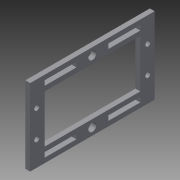
# Autodesk Inventor part: Motor_Mount_Side
Saved by Autodesk Inventor 2014 SP1 (Build 180222100, 222)
## iProperties
Created: 2014-03-20
Part Number: Motor_Mount_Side
Material: Generic
Document SubType Name: Modeling
Designer: ehagerup
Density: 1 g/cm^3
Appearance: Default
Author: ehagerup
Autodesk Inventor part; units mm, degrees
ref_plane "YZ Plane" through (0, 0, 0) normal (1, 0, 0) x (0, 1, 0)
ref_plane "XZ Plane" through (0, 0, 0) normal (0, 1, 0) x (-1, 0, 0)
ref_plane "XY Plane" through (0, 0, 0) normal (0, 0, 1) x (1, 0, 0)
sketch "Sketch1" plane through (0, 0, 0) normal (1, 0, 0) x (0, 1, 0)
  line L0 (0, 0) -> (60, 0)
  line L1 (60, 0) -> (60, 30)
  line L2 (60, 30) -> (0, 30)
  line L3 (0, 30) -> (0, 0)
  line L4 (-9, -9) -> (69, -9)
  line L5 (69, -9) -> (69, 39)
  line L6 (69, 39) -> (-9, 39)
  line L7 (-9, 39) -> (-9, -9)
  circle A0 centre (64.8, 23.5) radius 1.6
  circle A1 centre (64.8, 6.5) radius 1.6
  circle A2 centre (-4.8, 23.5) radius 1.6
  circle A3 centre (-4.8, 6.5) radius 1.6
  line L8 (0, 33) -> (20, 33)
  line L9 (20, 33) -> (20, 36)
  line L10 (20, 36) -> (0, 36)
  line L11 (0, 36) -> (0, 33)
  line L12 (60, 33) -> (40, 33)
  line L13 (40, 33) -> (40, 36)
  line L14 (40, 36) -> (60, 36)
  line L15 (60, 36) -> (60, 33)
  circle A4 centre (30, 34.5) radius 2.5
  circle A5 centre (30, -4.5) radius 2.5
  line L16 (0, -3) -> (20, -3)
  line L17 (20, -3) -> (20, -6)
  line L18 (20, -6) -> (0, -6)
  line L19 (0, -6) -> (0, -3)
  line L20 (60, -3) -> (40, -3)
  line L21 (40, -3) -> (40, -6)
  line L22 (40, -6) -> (60, -6)
  line L23 (60, -6) -> (60, -3)
  dimension "d0" = 60
  dimension "d1" = 30
  dimension "d2" = 4.8
  dimension "d3" = 4.8
  dimension "d4" = 4.8
  dimension "d5" = 4.8
  dimension "d6" = 3.2
  dimension "d7" = 3.2
  dimension "d8" = 3.2
  dimension "d9" = 3.2
  dimension "d10" = 6.5
  dimension "d11" = 6.5
  dimension "d12" = 6.5
  dimension "d13" = 6.5
  dimension "d14" = 9
  dimension "d15" = 9
  dimension "d16" = 9
  dimension "d17" = 9
  dimension "d18" = 20
  dimension "d19" = 9
  dimension "d20" = 3
  dimension "d21" = 3
  dimension "d22" = 9
  dimension "d23" = 3
  dimension "d24" = 3
  dimension "d25" = 20
  dimension "d26" = 5
  dimension "d27" = 10
  dimension "d28" = 4.5
  dimension "d29" = 4.5
  dimension "d30" = 5
  dimension "d31" = 3
  dimension "d32" = 3
  dimension "d33" = 20
  dimension "d34" = 9
  dimension "d35" = 10
  dimension "d36" = 10
  dimension "d37" = 20
  dimension "d38" = 3
  dimension "d39" = 3
  constraints: 48 end point, 12 parallel, 6 centre point, 6 horizontal, 6 perpendicular
  measures "d0" distance of L1.end L2.end
  measures "d1" distance of L0.end L1.end
  measures "d2" distance from line of A1.centre L1
  measures "d3" distance from line of A0.centre L1
  measures "d4" distance from line of L3 A2.centre
  measures "d5" distance from line of L3 A3.centre
  measures "d6" diameter of A1
  measures "d7" diameter of A0
  measures "d8" diameter of A3
  measures "d9" diameter of A2
  measures "d10" distance from line of L2 A2.centre
  measures "d11" distance from line of L0 A3.centre
  measures "d12" distance from line of L0 A1.centre
  measures "d13" distance from line of L2 A0.centre
  measures "d14" distance between parallel lines of L6 L2
  measures "d15" distance between parallel lines of L4 L0
  measures "d16" distance between parallel lines of L7 L3
  measures "d17" distance between parallel lines of L1 L5
  measures "d18" distance of L13.end L14.end
  measures "d19" distance between parallel lines of L5 L15
  measures "d20" distance between parallel lines of L2 L12
  measures "d21" distance between parallel lines of L14 L12
  measures "d22" distance between parallel lines of L7 L11
  measures "d23" distance between parallel lines of L2 L8
  measures "d24" distance between parallel lines of L6 L10
  measures "d25" distance between parallel lines of L11 L9
  measures "d26" diameter of A4
  measures "d27" distance from line of L13 A4.centre
  measures "d28" distance from line of L6 A4.centre
  measures "d29" distance from line of L0 A5.centre
  measures "d30" diameter of A5
  measures "d31" distance between parallel lines of L0 L20
  measures "d32" distance between parallel lines of L20 L22
  measures "d33" distance of L20.start L20.end
  measures "d34" distance between parallel lines of L5 L23
  measures "d35" distance from line of L21 A5.centre
  measures "d36" distance from line of A5.centre L17
  measures "d37" distance of L16.start L16.end
  measures "d38" distance between parallel lines of L0 L16
  measures "d39" distance between parallel lines of L18 L16
extrude "Extrusion1" add sketch "Sketch1" along normal blind 3
body "Solid1"
